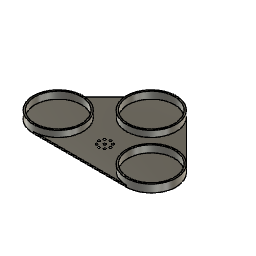
工训赛物流小车载物台 v3 (Autodesk Fusion 360 design; units mm, degrees)
Autodesk Fusion 360 part; units mm, degrees
note: some values were not read from the file. Set by a fixed rule: which sketch regions a step uses.
sketch "草图1" plane through (0, 0, 0) normal (0, 1, 0) x (1, 0, 0)
  circle A0 centre (6.053, -99.8166) radius 30
  circle A1 centre (89.4703, -44.6663) radius 30
  circle A2 centre (-83.4172, -55.1504) radius 30
  line L0 (-27.4834, -7.8873) -> (-91.6927, -26.3144)
  line L1 (28.2351, -4.5085) -> (94.2006, -15.0415)
  arc A3 (-108.4424, -71.6955) -> (116.3113, -58.0661) centre (0, 0) ccw
  arc A4 (116.3113, -58.0661) -> (94.2006, -15.0415) centre (89.4703, -44.6663) ccw
  arc A5 (-91.6927, -26.3144) -> (-108.4424, -71.6955) centre (-83.4172, -55.1504) ccw
  arc A6 (19.9701, 3.5948) -> (-20.2582, 1.1553) centre (0, 0) ccw
  arc A7 (-27.4834, -7.8873) -> (-20.2582, 1.1553) centre (-30.2419, 1.7247) ccw
  arc A8 (19.9701, 3.5948) -> (28.2351, -4.5085) centre (29.8119, 5.3664) ccw
  circle A9 centre (-83.4172, -55.1504) radius 28
  circle A10 centre (89.4703, -44.6663) radius 28
  circle A11 centre (6.053, -99.8166) radius 28
  dimension "d2" = 60
  dimension "d4" = 360
  dimension "d5" = 30
  dimension "d6" = 30
  dimension "d7" = 10
  dimension "d8" = -2
  dimension "d9" = -2
  dimension "d10" = -2
  constraint coincident A3.centre A6.centre
  constraint tangent A0 A3
  constraint tangent A2 L0
  constraint tangent A1 L1
  constraint tangent L1 A4
  constraint tangent A3 A4
  constraint tangent L0 A5
  constraint tangent A3 A5
  constraint concentric A3 A6
  constraint tangent L0 A7
  constraint tangent A6 A7
  constraint tangent A6 A8
  constraint tangent L1 A8
  constraint equal A7 A8
  measures "d2" diameter of A0
  measures "d5" radius of A4
  measures "d6" radius of A5
  measures "d7" radius of A7
sketch "草图2" plane through (0, 0, 0) normal (0, 1, 0) x (-1, 0, 0)
  line L0 (27.4834, 7.8873) -> (91.6927, 26.3144)
  arc A0 (91.6927, 26.3144) -> (108.4424, 71.6955) centre (83.4172, 55.1504) ccw
  arc A1 (108.4424, 71.6955) -> (-116.3113, 58.0661) centre (0, 0) ccw
  arc A2 (-116.3113, 58.0661) -> (-94.2006, 15.0415) centre (-89.4703, 44.6663) ccw
  line L1 (-94.2006, 15.0415) -> (-28.2351, 4.5085)
  arc A3 (-19.9701, -3.5948) -> (-28.2351, 4.5085) centre (-29.8119, -5.3664) ccw
  arc A4 (-19.9701, -3.5948) -> (20.2582, -1.1553) centre (0, 0) ccw
  arc A5 (27.4834, 7.8873) -> (20.2582, -1.1553) centre (30.2419, -1.7247) ccw
sketch "草图3" plane through (0, 0, 0) normal (0, 1, 0) x (1, 0, 0)
  line L0 (-30, 350) -> (-60, 350)
  line L1 (21.2132, 268.7868) -> (81.2132, 328.7868)
  line L2 (-21.2132, 268.7868) -> (-81.2132, 328.7868)
  line L3 (60, 380) -> (-60, 380)
  arc A0 (-60, 380) -> (-81.2132, 328.7868) centre (-60, 350) ccw
  arc A1 (-21.2132, 268.7868) -> (21.2132, 268.7868) centre (0, 290) ccw
  arc A2 (81.2132, 328.7868) -> (60, 380) centre (60, 350) ccw
  arc A3 (-60, 382) -> (-82.6274, 327.3726) centre (-60, 350) ccw
  line L4 (-22.6274, 267.3726) -> (-82.6274, 327.3726)
  arc A4 (-22.6274, 267.3726) -> (22.6274, 267.3726) centre (0, 290) ccw
  line L5 (22.6274, 267.3726) -> (82.6274, 327.3726)
  arc A5 (82.6274, 327.3726) -> (60, 382) centre (60, 350) ccw
  line L6 (60, 382) -> (-60, 382)
  dimension "d25" = 60
  dimension "d26" = 60
  dimension "d27" = 60
  dimension "d28" = -2
  constraint coincident L0.end A0.centre
  constraint tangent L1 A2
  constraint tangent L1 A1
  measures "d25" diameter of A1
  measures "d26" diameter of A2
  measures "d27" diameter of A0
extrude "拉伸4" add sketch "草图3" along normal blind 2 contours L1 L2 L3 A0 A1 A2 | A3 L4 A4 L5 A5 L6
sketch "草图4" plane through (0, 0, 0) normal (0, 1, 0) x (1, 0, 0)
  circle A0 centre (-60, 350) radius 30
  circle A1 centre (0, 290) radius 30
  circle A2 centre (60, 350) radius 30
  circle A3 centre (0, 290) radius 32
  circle A4 centre (-60, 350) radius 32
  circle A5 centre (60, 350) radius 32
  dimension "d31" = 60
  dimension "d32" = 60
  dimension "d33" = 60
  dimension "d34" = 2
  dimension "d35" = 2
  dimension "d36" = 2
  measures "d31" diameter of A0
  measures "d32" diameter of A1
  measures "d33" diameter of A2
extrude "拉伸5" add sketch "草图4" against normal blind 20
sketch "草图5" plane through (0, 0, 0) normal (0, 1, 0) x (1, 0, 0)
  line L0 (-60, 350) -> (60, 350)
  line L1 (0, 290) -> (0, 370)
  circle A0 centre (0, 350) radius 1.5
  line L2 (0, 350) -> (-10, 350)
  line L3 (0, 350) -> (-7.5, 350)
  circle A1 centre (-7.5, 350) radius 1.5
  circle A2 centre (-5.3033, 344.6967) radius 1.5
  circle A3 centre (0, 342.5) radius 1.5
  circle A4 centre (5.3033, 344.6967) radius 1.5
  circle A5 centre (7.5, 350) radius 1.5
  circle A6 centre (5.3033, 355.3033) radius 1.5
  circle A7 centre (0, 357.5) radius 1.5
  circle A8 centre (-5.3033, 355.3033) radius 1.5
  point P0 (-10, 350)
  dimension "d39" = 3
  dimension "d40" = 7.5
  dimension "d41" = 3
  dimension "d43" = 360
  constraint horizontal L0
  constraint perpendicular L0 L1
  constraint midpoint L0 A0.centre
  constraint coincident A0.centre L2.start
  constraint coincident L0 P0
  constraint perpendicular L1 L2
  constraint coincident P0 L2.end
  constraint parallel L0 L3
  constraint coincident L3.end A1.centre
  measures "d39" diameter of A0
  measures "d40" distance of A0.centre L3.end
  measures "d41" diameter of A1
extrude "拉伸6" cut sketch "草图5" along normal mid plane 20
move_body "移动1" bodies 1 to x (1, 0, 0) y (0, 0, -1) z (0, 1, 0) at (0, 330, -370)
extrude "拉伸7" cut 3 faces at (31.2142, 41.5898, -350) (-28.8975, -16.9198, -350) (91.2142, -18.4102, -350) along direction (0, 0, -1) blind 10
sketch "草图6" plane through (0, 0, 0) normal (0, 1, 0) x (1, 0, 0)
extrude "拉伸8" cut 3 faces at (31.2142, 41.5898, -360) (-28.8975, -16.9198, -360) (91.2142, -18.4102, -360) along direction (0, 0, -1) blind 2
extrude "拉伸9" cut 3 faces at (-54.9184, -29.7493, -370) (3.6534, 30.6913, -370) (59.203, -29.3087, -370) along direction (0, 0, -1) blind 1
